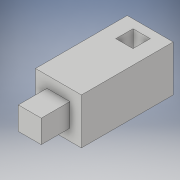
# Autodesk Inventor part: SquareCrank_SBail
Saved by Autodesk Inventor 2019 (Build 230136000, 136)
## iProperties
Created: 2019-05-06
Part Number: SquareCrank_SBail
Material: Generic
Document SubType Name: Modeling
Designer: samson.bailor
Density: 1 g/cm^3
Appearance: Default
Author: samson.bailor
Autodesk Inventor part; units mm, degrees
ref_plane "YZ Plane" through (0, 0, 0) normal (1, 0, 0) x (0, 1, 0)
ref_plane "XZ Plane" through (0, 0, 0) normal (0, 1, 0) x (-1, 0, 0)
ref_plane "XY Plane" through (0, 0, 0) normal (0, 0, 1) x (1, 0, 0)
sketch "Sketch1" plane through (0, 0, 0) normal (0, 0, 1) x (1, 0, 0)
  line L0 (0, 0) -> (50.8, 0)
  line L1 (50.8, 0) -> (50.8, 50.8)
  line L2 (50.8, 50.8) -> (0, 50.8)
  line L3 (0, 50.8) -> (0, 0)
  dimension "d0" = 50.8
  dimension "d1" = 50.8
  constraints: 8 end point, 2 parallel, 1 horizontal, 1 perpendicular
  measures "d0" distance of L2.end L1.end
  measures "d1" distance of L1.end L0.end
extrude "Extrusion1" add sketch "Sketch1" along normal blind 101.6
sketch "Sketch2" plane through (0, 0, 101.6) normal (0, 0, 1) x (1, 0, 0)
  line L0 (50.8, 50.8) -> (0, 50.8) projected
  line L1 (25.4, 38.1) -> (12.7, 38.1)
  line L2 (12.7, 38.1) -> (38.1, 38.1)
  line L3 (38.1, 38.1) -> (38.1, 12.7)
  line L4 (38.1, 12.7) -> (12.7, 12.7)
  line L5 (12.7, 12.7) -> (12.7, 38.1)
  point P0 (0, 0)
  dimension "d8" = 25.4
  dimension "d9" = 25.4
  constraints: 10 end point, 2 horizontal, 2 parallel, 1 perpendicular
  measures "d8" distance of L3.end L4.end
  measures "d9" distance of L2.end L3.end
extrude "Extrusion2" add sketch "Sketch2" along normal blind 31.75
sketch "Sketch3" plane through (0, 50.8, 0) normal (0, 1, 0) x (1, 0, 0)
  line L0 (50.8, 0) -> (0, 0) projected
  line L1 (25.4, 0) -> (25.4, -25.4)
  line L2 (25.4, -25.4) -> (19.05, -25.4)
  line L3 (19.05, -25.4) -> (19.05, -12.7)
  line L4 (19.05, -12.7) -> (25.4, -12.7)
  line L5 (25.4, -12.7) -> (25.4, -25.4)
  line L6 (25.4, -25.4) -> (31.75, -25.4)
  line L7 (31.75, -25.4) -> (31.75, -12.7)
  line L8 (31.75, -12.7) -> (25.4, -12.7)
  line L9 (25.4, -12.7) -> (25.4, -25.4)
  dimension "d12" = 25.4
  dimension "d13" = 6.35
  dimension "d14" = 12.7
  dimension "d15" = 6.35
  constraints: 18 end point, 4 parallel, 2 horizontal, 2 perpendicular, 1 midpoint, 1 point on line, 1 vertical
  measures "d12" distance of L1.start L1.end
  measures "d13" distance of L3.end L4.end
  measures "d14" distance of L2.end L3.end
  measures "d15" distance of L8.end L7.end
extrude "Extrusion3" cut sketch "Sketch3" against normal blind 25.4
sketch "Sketch4" plane through (0, 50.8, 0) normal (0, 1, 0) x (1, 0, 0)
  line L0 (19.05, -25.4) -> (19.05, -12.7) projected
  line L1 (19.05, -19.05) -> (15.875, -19.05)
  line L2 (0, 0) -> (0, -101.6) projected
  line L3 (15.875, -19.05) -> (34.925, -19.05)
  line L4 (34.925, -19.05) -> (34.925, -28.575)
  line L5 (34.925, -28.575) -> (15.875, -28.575)
  line L6 (15.875, -28.575) -> (15.875, -19.05)
  line L7 (34.925, -19.05) -> (15.875, -19.05)
  line L8 (15.875, -19.05) -> (15.875, -9.525)
  line L9 (15.875, -9.525) -> (34.925, -9.525)
  line L10 (34.925, -9.525) -> (34.925, -19.05)
  dimension "d18" = 3.175
  dimension "d19" = 19.05
  dimension "d20" = 9.525
  dimension "d21" = 19.05
  dimension "d22" = 9.525
  constraints: 18 end point, 4 parallel, 3 perpendicular, 2 horizontal, 1 midpoint
  measures "d18" distance of L1.start L1.end
  measures "d19" distance of L4.end L5.end
  measures "d20" distance of L3.end L4.end
  measures "d21" distance of L8.end L9.end
  measures "d22" distance of L7.end L8.end
extrude "Extrusion4" cut sketch "Sketch4" against normal blind 25.4
body "Solid1"
